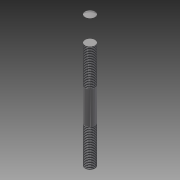
# Autodesk Inventor part: Oś piasty
Saved by Autodesk Inventor 2015 (Build 190159000, 159)
## iProperties
Created: 2015-11-24
Part Number: Oś piasty
Material: Aluminium AW-7020
Document SubType Name: Modeling
Designer: graaapsik
Density: 2.78 g/cm^3
Appearance: Aluminium AW-7020
Mass: 60.0553 g
Surface Area: 76.215 cm^2
Volume: 21.6026 cm^3
Author: graaapsik
Autodesk Inventor part; units mm, degrees
ref_plane "YZ Plane" through (0, 0, 0) normal (1, 0, 0) x (0, 1, 0)
ref_plane "XZ Plane" through (0, 0, 0) normal (0, 1, 0) x (-1, 0, 0)
ref_plane "XY Plane" through (0, 0, 0) normal (0, 0, 1) x (1, 0, 0)
sketch "Szkic1" plane through (0, 0, 0) normal (0, 0, 1) x (1, 0, 0)
  circle A0 centre (0, 0) radius 6
  dimension "d0" = 12
  constraints: 1 centre point, 1 coincident
  measures "d0" diameter of A0
extrude "Oś" add sketch "Szkic1" along normal blind 90 and the other way blind 100
thread "Gwint1" size "M12x1.75" class "6g" standard "ISO Metric profile" length 45
thread "Gwint2" size "M12x1.75" class "6g" standard "ISO Metric profile" length 45
sketch "Szkic4" plane through (0, 0, 0) normal (0, 1, 0) x (-1, 0, 0)
  arc A0 (-6, -100) -> (0, -101) centre (0, -82.5) ccw
  line L0 (0, 0) -> (5.8281, -2.2004) construction
  line L1 (-6, -100) -> (6, -100) construction
  line L2 (0, -100) -> (-6, -100)
  line L3 (0, -100) -> (0, -101)
  line L4 (0, 0) -> (7.1685, 0) construction
  arc A1 (0, 101) -> (-6, 100) centre (0, 82.5) ccw
  line L5 (-6, 100) -> (6, 100) construction
  line L6 (0, 100) -> (-6, 100)
  line L7 (0, 100) -> (0, 101)
  point P0 (4.76, -82.5)
  dimension "d21" = 1
  constraints: 14 end point, 5 symmetric about line, 4 point on circle, 2 centre point, 2 perpendicular, 1 horizontal, 1 line through centre, 3 other
  measures "d21" distance of L2.start L3.end
revolve "Obrót zakończeń" add sketch "Szkic4" angle 360 about axis through (0, 0, -100) along (0, 0, -1)
